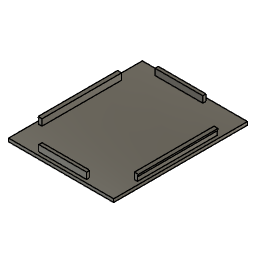
Lora Base Case Deckel (Autodesk Fusion 360 design; units mm, degrees)
Autodesk Fusion 360 part; units mm, degrees
sketch "Skizze1" plane through (0, 0, 0) normal (0, 0, 1) x (1, 0, 0)
  line L0 (-30, 35) -> (32, 35)
  line L1 (32, 35) -> (32, -45)
  line L2 (32, -45) -> (-30, -45)
  line L3 (-30, -45) -> (-30, 35)
  line L4 (34, 37) -> (34, -47)
  line L5 (34, -47) -> (-32, -47)
  line L6 (-32, -47) -> (-32, 37)
  line L7 (-32, 37) -> (34, 37)
  dimension "d1" = 62
  dimension "d2" = 80
  dimension "d3" = -2
  constraint horizontal L0
  constraint vertical L1
  constraint horizontal L2
  constraint vertical L3
  measures "d1" distance of L0.start L0.end
  measures "d2" distance of L0.end L1.end
  measures "d7" distance of L0.start
  measures "d8" distance of L0.start
  measures "d9" distance of L0.start
extrude "Extrusion1" add sketch "Skizze1" along normal blind 2 contours L0 L1 L2 L3 | L4 L5 L6 L7
sketch "Skizze2" plane through (0, 0, 2) normal (0, 0, 1) x (-1, 0, 0)
  line L0 (32, -37) -> (32, 47)
  line L1 (32, 47) -> (-34, 47)
  line L2 (-34, 47) -> (-34, -37)
  line L3 (-34, -37) -> (32, -37)
  line L4 (-32, 45) -> (-32, -35)
  line L5 (-32, -35) -> (30, -35)
  line L6 (30, -35) -> (30, 45)
  line L7 (30, 45) -> (-32, 45)
  line L8 (30, -20) -> (28, -20)
  line L9 (28, -20) -> (28, 30)
  line L10 (28, 30) -> (30, 30)
  line L11 (30, 30) -> (30, -20)
  line L12 (-32, -20) -> (-30, -20)
  line L13 (-30, -20) -> (-30, 30)
  line L14 (-30, 30) -> (-32, 30)
  line L15 (-32, 30) -> (-32, -20)
  line L16 (15, 45) -> (-15, 45)
  line L17 (-15, 45) -> (-15, 43)
  line L18 (-15, 43) -> (15, 43)
  line L19 (15, 43) -> (15, 45)
  line L20 (20, -35) -> (-10, -35)
  line L21 (-10, -35) -> (-10, -33)
  line L22 (-10, -33) -> (20, -33)
  line L23 (20, -33) -> (20, -35)
  dimension "d6" = -2
  dimension "d7" = 2
  dimension "d8" = 50
  dimension "d9" = 15
  dimension "d10" = 50
  dimension "d11" = 15
  dimension "d12" = 2
  dimension "d16" = 2
  dimension "d17" = 2
  dimension "d18" = 30
  dimension "d19" = 30
  dimension "d21" = 15
  dimension "d28" = 10
  constraint horizontal L8
  constraint vertical L9
  constraint horizontal L10
  constraint vertical L11
  constraint coincident L6 L8.start
  constraint horizontal L12
  constraint vertical L13
  constraint horizontal L14
  constraint vertical L15
  constraint coincident L4 L12.start
  constraint horizontal L16
  constraint vertical L17
  constraint horizontal L18
  constraint vertical L19
  constraint coincident L7 L16.start
  constraint horizontal L20
  constraint vertical L21
  constraint horizontal L22
  constraint vertical L23
  constraint coincident L5 L20.start
  measures "d7" distance of L8.start L8.end
  measures "d8" distance of L8.end L9.end
  measures "d9" distance of L5 L8.end
  measures "d10" distance of L12.end L13.end
  measures "d11" distance of L5 L12.end
  measures "d12" distance of L12.start L12.end
  measures "d16" distance of L20.end L21.end
  measures "d17" distance of L16.end L17.end
  measures "d18" distance of L21.end L22.end
  measures "d19" distance of L17.end L18.end
  measures "d21" distance of L6 L19
  measures "d28" distance of L6 L23
extrude "Extrusion2" add sketch "Skizze2" along normal blind 4 contours L4 L12 L13 L14 L15 | L7 L16 L17 L18 L19 | L5 L20 L21 L22 L23 | L6 L8 L9 L10 L11
sketch "Skizze5" plane through (32, 0, 0) normal (1, 0, 0) x (0, 1, 0)
  line L0 (-30, 2) -> (20, 2)
  line L1 (20, 2) -> (20, 6)
  line L2 (20, 6) -> (-30, 6)
  line L3 (-30, 6) -> (-30, 2)
  line L4 (-30, 5) -> (20, 5)
  dimension "d29" = 1
  constraint coincident L3 L4.start
  constraint coincident L1 L4.end
  constraint perpendicular L1 L4
  measures "d29" distance of L2 L4
extrude "Extrusion5" add sketch "Skizze5" along normal blind 0.5 contours L1 L2 L3 L4
sketch "Skizze6" plane through (-30, 0, 0) normal (-1, 0, 0) x (0, -1, 0)
  line L0 (-20, 2) -> (30, 2)
  line L1 (30, 2) -> (30, 6)
  line L2 (30, 6) -> (-20, 6)
  line L3 (-20, 6) -> (-20, 2)
  line L4 (-20, 5) -> (30, 5)
  dimension "d32" = 1
  constraint coincident L3 L4.start
  constraint coincident L1 L4.end
  constraint perpendicular L1 L4
  measures "d32" distance of L2 L4
extrude "Extrusion6" add sketch "Skizze6" along normal blind 0.5 contours L1 L2 L3 L4
